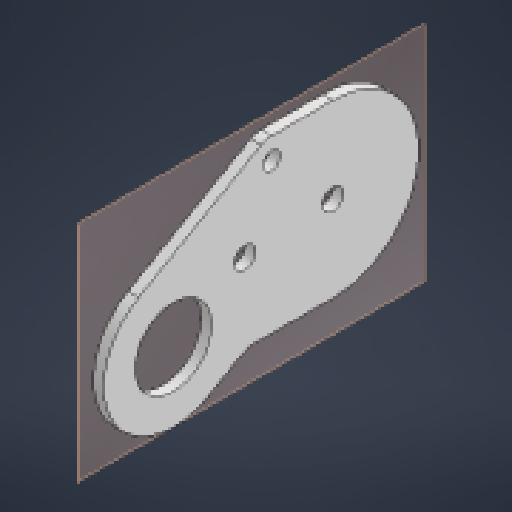
# Autodesk Inventor part: DCX16_Mount
Saved by Autodesk Inventor 2024.2 (Build 282272000, 272)
## iProperties
Created: 2024-02-18
Part Number: DCX16_Mount
Material: 一般
Document SubType Name: Modeling
Designer: Hanaoka
Density: 1 g/cm^3
Appearance: 既定
Author: Hanaoka
Autodesk Inventor part; units mm, degrees
ref_plane "YZ Plane" through (0, 0, 0) normal (1, 0, 0) x (0, 1, 0)
ref_plane "XZ Plane" through (0, 0, 0) normal (0, 1, 0) x (-1, 0, 0)
ref_plane "XY Plane" through (0, 0, 0) normal (0, 0, 1) x (1, 0, 0)
ref_plane "作業平面1" through (4.373, -15.3402, 16.1739) normal (1, 0, 0) x (0, 1, 0)
sketch "スケッチ1" plane through (4.373, -15.3402, 16.1739) normal (1, 0, 0) x (0, 1, 0)
  circle A0 centre (0, 0) radius 3.6 projected
  circle A1 centre (4.4971, -14.9328) radius 1 projected
  circle A2 centre (3.8857, -6.7055) radius 1 projected
  circle A3 centre (10.4971, -9.1815) radius 0.8 projected
  arc A4 (-3.5029, -14.9328) -> (12.4971, -14.9328) centre (4.4971, -14.9328) ccw projected
  line L0 (12.4971, -14.9328) -> (12.4971, -9.1815) projected
  arc A5 (12.4971, -9.1815) -> (12.2292, -8.1815) centre (10.4971, -9.1815) ccw projected
  line L1 (12.2292, -8.1815) -> (5.6292, 3.25) projected
  arc A6 (5.6292, 3.25) -> (-5.6292, -3.25) centre (0, 0) ccw projected
  line L2 (-5.6292, -3.25) -> (-3.9048, -6.2367) projected
  arc A7 (-3.5029, -7.7367) -> (-3.9048, -6.2367) centre (-6.5029, -7.7367) ccw projected
  line L3 (-3.5029, -7.7367) -> (-3.5029, -14.9328) projected
  point P0 (15.3402, -16.1739)
extrude "押し出し1" add sketch "スケッチ1" along normal blind 1
